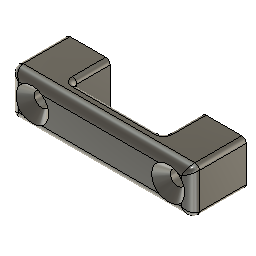
agraphe_bande_leds v4 (Autodesk Fusion 360 design; units mm, degrees)
Autodesk Fusion 360 part; units mm, degrees
sketch "Esquisse1" plane through (0, 0, 0) normal (0, 1, 0) x (1, 0, 0)
  line L0 (20.25, 5) -> (-20.25, 5)
  line L1 (-20.25, 5) -> (-20.25, -5)
  line L2 (-20.25, -5) -> (20.25, -5)
  line L3 (20.25, -5) -> (20.25, 5)
  line L4 (20.25, 5) -> (-20.25, -5) construction
  line L5 (-20.25, 5) -> (20.25, -5) construction
  dimension "d1" = 40.5
  dimension "d2" = 10
  constraint horizontal L0
  constraint perpendicular L0 L1
  constraint parallel L0 L2
  constraint parallel L1 L3
  constraint coincident L4 origin
  constraint coincident L5 origin
  measures "d1" distance of L1.end L2.end
  measures "d2" distance of L0.end L1.end
extrude "Extrusion1" add sketch "Esquisse1" along normal blind 4
sketch "Esquisse5" plane through (0, 0, 0) normal (0, 1, 0) x (1, 0, 0)
  line L0 (-10.25, 5) -> (-20.25, 5)
  line L1 (-20.25, 5) -> (-20.25, -5)
  line L2 (-20.25, -5) -> (-10.25, -5)
  line L3 (-10.25, -5) -> (-10.25, 5)
  line L4 (-10.25, 5) -> (-20.25, -5) construction
  line L5 (-20.25, 5) -> (-10.25, -5) construction
  circle A0 centre (-15.25, 0) radius 1.6
  line L6 (20.25, 5) -> (-20.25, 5)
  point P0 (-15.25, 0)
  dimension "d26" = 10
  dimension "d27" = 10
  dimension "d28" = 15.25
  dimension "d29" = 3.2
  dimension "d46" = 5
  constraint horizontal L0
  constraint perpendicular L0 L1
  constraint parallel L0 L2
  constraint parallel L1 L3
  constraint coincident L4 P0
  constraint coincident L5 P0
  constraint coincident P0 A0.centre
  measures "d26" distance of L1.end L2.end
  measures "d27" distance of L0.end L1.end
  measures "d28" distance of P0 origin
  measures "d29" diameter of A0
  measures "d46" distance of P0 L6
extrude "Extrusion7" add sketch "Esquisse5" along normal blind 12.5
extrude "Extrusion8" cut sketch "Esquisse5" along normal blind 4 contours A0
sketch "Esquisse6" plane through (0, 0, 0) normal (0, 1, 0) x (1, 0, 0)
  line L0 (20.25, -5) -> (20.25, 5)
  line L1 (10.25, 5) -> (20.25, -5) construction
  line L2 (10.25, 5) -> (10.25, -5)
  line L3 (20.25, 5) -> (10.25, 5)
  line L4 (10.25, -5) -> (20.25, -5)
  circle A0 centre (15.25, 0) radius 1.6
  line L5 (20.25, 5) -> (10.25, -5) construction
  line L6 (20.25, 5) -> (-20.25, 5)
  point P0 (15.25, 0)
  point P1 (28, 0)
  point P2 (28, 0)
  dimension "d34" = 10
  dimension "d35" = 10
  dimension "d37" = 3.2
  dimension "d38" = 15.25
  dimension "d47" = 5
  constraint horizontal L3
  constraint perpendicular L2 L3
  constraint parallel L3 L4
  constraint parallel L0 L2
  constraint coincident P0 L5
  constraint coincident P0 L1
  constraint coincident P0 A0.centre
  measures "d34" distance of L2.end L0.start
  measures "d35" distance of L1.start L2.end
  measures "d37" diameter of A0
  measures "d38" distance of P0 origin
  measures "d47" distance of P0 L6
extrude "Extrusion9" add sketch "Esquisse6" along normal blind 12.5
extrude "Extrusion10" cut sketch "Esquisse6" along normal blind 4 contours A0
chamfer "Chanfrein3" distance 2.1 angle 45 2 edges at (-16.7417, 0, 0.5786) (13.7583, 0, 0.5786)
sketch "Esquisse8" plane through (0, 4, 0) normal (0, 1, 0) x (-1, 0, 0)
  line L0 (-10.25, 5) -> (-10.25, -5)
  line L1 (-10.25, -5) -> (10.25, -5)
  line L2 (10.25, -5) -> (10.25, 5)
  line L3 (10.25, 5) -> (-10.25, 5)
  line L4 (8.25, -3) -> (-8.25, -3)
  line L5 (-8.25, -3) -> (-8.25, 3)
  line L6 (-8.25, 3) -> (8.25, 3)
  line L7 (8.25, 3) -> (8.25, -3)
  line L8 (8.25, -3) -> (-8.25, 3) construction
  line L9 (-8.25, -3) -> (8.25, 3) construction
  dimension "d52" = 16.5
  dimension "d53" = 6
  constraint horizontal L4
  constraint perpendicular L4 L5
  constraint parallel L4 L6
  constraint parallel L5 L7
  constraint coincident L8 origin
  constraint coincident L9 origin
  measures "d52" distance of L5.end L6.end
  measures "d53" distance of L4.end L5.end
extrude "Extrusion12" cut sketch "Esquisse8" against normal blind 2 contours L4 L5 L6 L7
fillet "Congé1" radius 1 2 edges at (-10.25, 4, 0) (10.25, 4, 0)
fillet "Congé2" radius 1 14 edges at (-10.25, 8.75, 5) (-9.9571, 4.2929, 5) (0, 4, 5) (9.9571, 4.2929, 5) (10.25, 8.75, 5) (10.25, 8.75, -5) (9.9571, 4.2929, -5) (0, 4, -5) (-9.9571, 4.2929, -5) (-10.25, 8.75, -5) (20.25, 6.25, 5) (-20.25, 6.25, -5) (20.25, 6.25, -5) (-20.25, 6.25, 5)
fillet "Congé3" radius 2 8 edges at (20.25, 0, 0) (19.9571, 0, -4.7071) (0, 0, -5) (-19.9571, 0, -4.7071) (-20.25, 0, 0) (-19.9571, 0, 4.7071) (0, 0, 5) (19.9571, 0, 4.7071)
fillet "Congé4" radius 1 6 edges at (0, 2, -3) (8.25, 2, 0) (-8.25, 2, 0) (0, 2, 3) (-8.25, 4, 0) (8.25, 4, 0)
equation "d1 = portée_pont + longueur_pile * 2"
equation "d2 = largeur_pont"
equation "d3 = epaisseur_pont"
equation "portée_pont = 20.5 mm"
equation "hauteur_pont = 8.5 mm"
equation "longueur_pile = vis_dia_tete + 3 mm"
equation "vis_dia_percage = 3.2 mm"
equation "epaisseur_pont = 4 mm"
equation "largeur_pont = vis_dia_tete + 3 mm"
equation "d26 = longueur_pile"
equation "d27 = largeur_pont"
equation "d28 = portée_pont / 2 + longueur_pile / 2"
equation "d29 = vis_dia_percage"
equation "d30 = epaisseur_pont + hauteur_pont"
equation "d32 = epaisseur_pont"
equation "d34 = longueur_pile"
equation "d35 = largeur_pont"
equation "d37 = vis_dia_percage"
equation "d38 = portée_pont / 2 + longueur_pile / 2"
equation "d39 = hauteur_pont + epaisseur_pont"
equation "d41 = epaisseur_pont"
equation "vis_dia_tete = 7 mm"
equation "d46 = largeur_pont / 2"
equation "d47 = largeur_pont / 2"
equation "d52 = portée_pont - 4 mm"
equation "d53 = largeur_pont - 4 mm"
equation "d54 = -epaisseur_pont + 2 mm"
equation "d58 = ( vis_dia_tete - vis_dia_percage ) / 2 + 0.2 mm"
